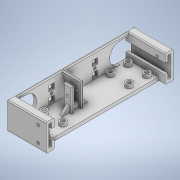
# Autodesk Inventor part: xEnd
Saved by Autodesk Inventor 2022 (Build 260153000, 153)
## iProperties
Created: 2020-01-28
Part Number: xEnd
Material: Generic
Document SubType Name: Modeling
Designer: PAB
Density: 1 g/cm^3
Appearance: Default
Author: PAB
Autodesk Inventor part; units mm, degrees
ref_plane "YZ Plane" through (0, 0, 0) normal (1, 0, 0) x (0, 1, 0)
ref_plane "XZ Plane" through (0, 0, 0) normal (0, 1, 0) x (-1, 0, 0)
ref_plane "XY Plane" through (0, 0, 0) normal (0, 0, 1) x (1, 0, 0)
sketch "Sketch1" plane through (0, 0, 0) normal (0, 1, 0) x (-1, 0, 0)
  line L0 (24, 94) -> (-24, 94)
  line L1 (-24, 94) -> (-24, -94)
  line L2 (-24, -94) -> (24, -94)
  line L3 (24, -94) -> (24, 94)
  point P0 (0, 0)
  dimension "d0" = 48
  dimension "d1" = 188
  constraints: 8 end point, 2 parallel, 1 horizontal, 1 perpendicular
  measures "d0" distance of L2.end L1.end
  measures "d1" distance of L1.end L0.end
extrude "Extrusion1" add sketch "Sketch1" along normal blind 5
sketch "Sketch2" plane through (0, 5, 0) normal (0, 1, 0) x (1, 0, 0)
  line L0 (24, -94) -> (24, 94) projected
  line L1 (-24, 94) -> (-24, -94) projected
  line L2 (24, -94) -> (-24, -94)
  line L3 (-24, -94) -> (-24, -90)
  line L4 (-24, -90) -> (24, -90)
  line L5 (24, -90) -> (24, -94)
  line L6 (24, 94) -> (-24, 94) projected
  line L7 (24, 94) -> (-24, 94)
  line L8 (-24, 94) -> (-24, 90)
  line L9 (-24, 90) -> (24, 90)
  line L10 (24, 90) -> (24, 94)
  line L11 (-24, 90) -> (-20, 90)
  line L12 (-20, 90) -> (-20, -90)
  line L13 (-20, -90) -> (-24, -90)
  line L14 (-24, -90) -> (-24, 90)
  line L15 (24, -30) -> (-20, -30)
  line L16 (-20, -30) -> (-20, -26)
  line L17 (-20, -26) -> (24, -26)
  line L18 (24, -26) -> (24, -30)
  line L19 (24, -16) -> (-20, -16)
  line L20 (-20, -16) -> (-20, -12)
  line L21 (-20, -12) -> (24, -12)
  line L22 (24, -12) -> (24, -16)
  point P0 (0, 0)
  point P1 (-20, -30)
  point P2 (24, -26)
  point P3 (-20, -16)
  point P4 (24, -12)
  dimension "d4" = 4
  dimension "d5" = 4
  dimension "d6" = 4
  dimension "d7" = 4
  dimension "d8" = 4
  dimension "d73" = 64
  dimension "d74" = 78
  constraints: 40 end point, 10 parallel, 7 point on line, 5 horizontal, 5 perpendicular
  measures "d4" distance of L2.end L3.end
  measures "d5" distance of L8.end L7.end
  measures "d6" distance of L12.end L13.end
  measures "d7" distance of L15.end L16.end
  measures "d8" distance of L19.end L20.end
  measures "d73" distance between parallel lines of L15 L2
  measures "d74" distance between parallel lines of L19 L2
extrude "Extrusion2" add sketch "Sketch2" along normal blind 35 contours L2 L1 L4 L0 | L15 L12 L17 L0 | L4 L1 L9 L12 | L1 L6 L0 L9 | L19 L12 L21 L0
sketch "Sketch3" plane through (-20, 5, 90) normal (1, 0, 0) x (0, 0, -1)
  line L0 (0, 0) -> (0, 35) projected
  line L1 (0, 35) -> (8, 35)
  line L2 (8, 35) -> (8, 31)
  line L3 (8, 31) -> (0, 31)
  line L4 (0, 31) -> (0, 35)
  line L5 (8, 31) -> (4, 31)
  line L6 (4, 31) -> (4, 23)
  line L7 (4, 23) -> (8, 23)
  line L8 (8, 23) -> (8, 31)
  line L9 (0, 0) -> (60, 0) projected
  line L10 (8, 0) -> (4, 0)
  line L11 (4, 0) -> (4, 8)
  line L12 (4, 8) -> (8, 8)
  line L13 (8, 8) -> (8, 0)
  line L14 (0, 35) -> (-4, 35)
  line L15 (-4, 35) -> (-4, -5)
  line L16 (-4, -5) -> (0, -5)
  line L17 (0, -5) -> (0, 35)
  line L18 (0, -5) -> (8, -5)
  line L19 (8, -5) -> (8, 0)
  line L20 (8, 0) -> (0, 0)
  line L21 (0, 0) -> (0, -5)
  point P0 (90, -5)
  point P1 (4, 0)
  point P2 (4, 31)
  dimension "d11" = 8
  dimension "d12" = 4
  dimension "d13" = 4
  dimension "d14" = 8
  dimension "d15" = 4
  dimension "d16" = 8
  constraints: 40 end point, 10 parallel, 5 horizontal, 5 perpendicular, 2 point on line
  measures "d11" distance of L2.end L3.end
  measures "d12" distance of L1.end L2.end
  measures "d13" distance of L7.end L6.end
  measures "d14" distance of L6.end L5.end
  measures "d15" distance of L11.end L12.end
  measures "d16" distance of L10.end L11.end
extrude "Extrusion3" add sketch "Sketch3" along normal blind 54
sketch "Sketch4" plane through (-20, 5, 30) normal (1, 0, 0) x (0, 0, -1)
  line L0 (-60, 0) -> (-60, 31) projected
  line L1 (-56, 8) -> (-56, 0) projected
  line L2 (-60, 31) -> (-56, 31)
  line L3 (-56, 31) -> (-56, 0)
  line L4 (-56, 0) -> (-60, 0)
  line L5 (-60, 0) -> (-60, 31)
  line L6 (-52, 23) -> (-56, 23) projected
  line L7 (-56, 8) -> (-52, 8) projected
  line L8 (-56, 23) -> (-52, 23)
  line L9 (-52, 23) -> (-52, 8)
  line L10 (-52, 8) -> (-56, 8)
  line L11 (-56, 8) -> (-56, 23)
  line L12 (-52, 35) -> (-52, 23) projected
  line L13 (0, 0) -> (-52, 0) projected
  line L14 (-52, 31) -> (-39.5, 31)
  line L15 (-39.5, 31) -> (-39.5, 0)
  line L16 (-39.5, 0) -> (-52, 0)
  line L17 (-52, 0) -> (-52, 31)
  arc A0 (-39.5, 0) -> (-39.5, 31) centre (-39.5, 15.5) ccw
  point P0 (30, -5)
  dimension "d19" = 12.5
  dimension "d20" = 15.5
  constraints: 24 end point, 6 parallel, 3 horizontal, 3 perpendicular, 3 point on line, 2 point on circle, 1 centre point
  measures "d19" distance of L15.end L16.end
  measures "d20" radius of A0
sketch "Sketch5" plane through (0, 5, 0) normal (0, 1, 0) x (1, 0, 0)
  circle A0 centre (14, -75) radius 3
  circle A1 centre (14, -49) radius 3
  circle A2 centre (-14, -75) radius 3
  circle A3 centre (-14, -49) radius 3
  point P0 (0, 0)
  dimension "d21" = 6
  dimension "d22" = 6
  dimension "d23" = 6
  dimension "d24" = 6
  constraints: 4 centre point
  measures "d21" diameter of A0
  measures "d22" diameter of A1
  measures "d23" diameter of A2
  measures "d24" diameter of A3
extrude "Extrusion4" cut sketch "Sketch5" against normal blind 54
sketch "Sketch6" plane through (0, 40, 0) normal (0, 1, 0) x (1, 0, 0)
  line L0 (-20, -30) -> (24, -30) projected
  line L1 (24, -12) -> (-20, -12) projected
  line L2 (24, -30) -> (24, -26) projected
  line L3 (24, -30) -> (8, -30)
  line L4 (8, -30) -> (8, -12)
  line L5 (8, -12) -> (24, -12)
  line L6 (24, -12) -> (24, -30)
  line L7 (24, -30) -> (-20, -30) projected
  line L8 (24, -16) -> (-20, -16) projected
  line L9 (-20, -30) -> (-4, -30)
  line L10 (-4, -30) -> (-4, -16)
  line L11 (-4, -16) -> (-20, -16)
  line L12 (-20, -16) -> (-20, -30)
  point P0 (0, 0)
  point P1 (24, -12)
  point P2 (8, -12)
  point P3 (8, -30)
  point P4 (-14, -52)
  point P5 (-20, -16)
  point P6 (-4, -30)
  dimension "d28" = 16
  dimension "d42" = 16
  constraints: 16 end point, 4 parallel, 2 horizontal, 2 perpendicular, 1 point on line, 2 other
  measures "d28" distance of L4.end L5.end
  measures "d42" distance of L11.end L10.end
extrude "Extrusion5" cut sketch "Sketch6" against normal blind 35 contours L12 L8 L10 L0 | L4 L8 L6 L2 L0 | L4 L1 L6 L8
sketch "Sketch7" plane through (0, 5, 0) normal (0, 1, 0) x (1, 0, 0)
  circle A0 centre (-14, -75) radius 3 projected
  circle A1 centre (-14, -75) radius 5
  circle A2 centre (-14, -49) radius 3 projected
  circle A3 centre (-14, -49) radius 5
  circle A4 centre (14, -49) radius 3 projected
  circle A5 centre (14, -49) radius 5
  circle A6 centre (14, -75) radius 3 projected
  circle A7 centre (14, -75) radius 5
  point P0 (0, 0)
  point P1 (-11.1716, -48)
  point P2 (-16.8284, -48)
  dimension "d31" = 10
  dimension "d32" = 10
  dimension "d33" = 10
  dimension "d34" = 10
  constraints: 4 centre point, 4 coincident
  measures "d31" diameter of A1
  measures "d32" diameter of A3
  measures "d33" diameter of A5
  measures "d34" diameter of A7
extrude "Extrusion6" add sketch "Sketch7" along normal blind 5
extrude "Extrusion7" cut sketch "Sketch4" against normal blind 5
sketch "Sketch8" plane through (8, 5, 12) normal (0, 0, -1) x (-1, 0, 0)
  circle A0 centre (6, 21.15) radius 2
  point P0 (8, -5)
  dimension "d49" = 4
  constraints: 1 centre point
  measures "d49" diameter of A0
sketch "Sketch9" plane through (-4, 5, 30) normal (0, 0, 1) x (1, 0, 0)
  line L0 (4, 0) -> (8, 0)
  line L1 (8, 0) -> (8, 10)
  line L2 (8, 10) -> (4, 10)
  line L3 (4, 10) -> (4, 0)
  point P0 (4, -5)
  dimension "d43" = 4
  dimension "d44" = 10
  constraints: 8 end point, 2 parallel, 1 horizontal, 1 perpendicular
  measures "d43" distance of L2.end L1.end
  measures "d44" distance of L1.end L0.end
extrude "Extrusion9" add sketch "Sketch9" along normal blind 10 and the other way blind 28
extrude "Extrusion10" cut sketch "Sketch8" against normal blind 18
sketch "Sketch10" plane through (4, 5, 12) normal (1, 0, 0) x (0, 0, -1)
  line L0 (-28, 10) -> (-28, 0) projected
  line L1 (-18, 10) -> (-28, 0)
  line L2 (-28, 0) -> (-28, 10)
  line L3 (-28, 10) -> (-18, 10)
  line L4 (10, 0) -> (10, 10) projected
  line L5 (10, 10) -> (0, 10) projected
  line L6 (10, 0) -> (0, 10)
  line L7 (10, 0) -> (10, 10)
  line L8 (10, 10) -> (0, 10)
  point P0 (12, -5)
  constraints: 13 end point, 2 perpendicular, 1 collinear, 1 vertical
extrude "Extrusion11" cut sketch "Sketch10" against normal blind 4
sketch "Sketch11" plane through (-20, 5, 12) normal (0, 0, -1) x (-1, 0, 0)
  line L0 (0, 0) -> (0, 35) projected
  line L1 (0, 31) -> (0, 0)
  line L2 (-16, 0) -> (-16, 35) projected
  line L3 (0, 0) -> (-16, 0)
  line L4 (-16, 0) -> (0, 31)
  point P0 (-20, -5)
  constraints: 6 end point, 1 collinear, 1 perpendicular, 1 point on line
extrude "Extrusion12" cut sketch "Sketch11" against normal blind 5
sketch "Sketch12" plane through (4, 5, 16) normal (1, 0, 0) x (0, 0, -1)
  line L0 (0, 10) -> (-10, 10) projected
  line L1 (0, 31) -> (0, 0) projected
  line L2 (-10, 10) -> (0, 10)
  line L3 (0, 10) -> (0, 7)
  line L4 (0, 7) -> (-10, 7)
  line L5 (-10, 7) -> (-10, 10)
  point P0 (16, -5)
  dimension "d56" = 3
  constraints: 8 end point, 2 parallel, 1 horizontal, 1 perpendicular, 1 point on line
  measures "d56" distance of L2.end L3.end
extrude "Extrusion13" cut sketch "Sketch12" against normal blind 5
sketch "Sketch13" plane through (-24, 0, 94) normal (0, 0, 1) x (1, 0, 0)
  circle A0 centre (46.5, 31) radius 2
  circle A1 centre (46.5, 8) radius 2
  line L0 (58, 40) -> (58, 0) projected
  point P0 (24, 0)
  dimension "d59" = 4
  dimension "d60" = 4
  dimension "d63" = 11.5
  dimension "d64" = 11.5
  constraints: 2 centre point
  measures "d59" diameter of A0
  measures "d60" diameter of A1
  measures "d63" distance from line of L0 A0.centre
  measures "d64" distance from line of L0 A1.centre
extrude "Extrusion14" cut sketch "Sketch13" against normal blind 12
sketch "Sketch14" plane through (-24, 0, -94) normal (-1, 0, 0) x (0, 0, 1)
  line L0 (130, 31) -> (122, 31)
  line L1 (122, 31) -> (122, 23)
  line L2 (122, 23) -> (130, 23)
  line L3 (130, 23) -> (130, 31)
  line L4 (130, 15) -> (122, 15)
  line L5 (122, 15) -> (122, 7)
  line L6 (122, 7) -> (130, 7)
  line L7 (130, 7) -> (130, 15)
  circle A0 centre (126, 19) radius 2
  point P0 (94, 0)
  dimension "d65" = 8
  dimension "d66" = 8
  dimension "d67" = 8
  dimension "d68" = 8
  dimension "d69" = 4
  constraints: 16 end point, 4 parallel, 2 horizontal, 2 perpendicular, 1 centre point, 1 point on line
  measures "d65" distance of L2.end L1.end
  measures "d66" distance of L1.end L0.end
  measures "d67" distance of L6.end L5.end
  measures "d68" distance of L5.end L4.end
  measures "d69" diameter of A0
extrude "Extrusion15" cut sketch "Sketch14" against normal blind 4
mirror "Mirror2" about plane through (0, 0, 0) normal (0, 0, 1) of "Extrusion15", "Extrusion14", "Extrusion7", "Extrusion6", "Extrusion4", "Extrusion3"
fillet "Fillet1" radius 1.5 24 edges at (-24, 40, 0) (5, 40, -94) (5, 40, 94) (7, 40, 82) (7, 40, -82) (5, 0, -94) (-24, 20, -94) (29, 0, 82) (5, 0, 94) (-24, 20, 94) (29, 0, -82) (-24, 0, 0) (-6, 40, 16) (-6, 40, 12) (2, 40, 30) (2, 40, 26) (-4, 22.5, 30) (-4, 22.5, 26) (8, 22.5, 30) (8, 22.5, 12) (8, 22.5, 16) (8, 22.5, 26) (-20, 40, -35) (-20, 40, 49)
body "Solid1"
